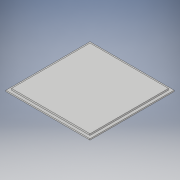
# Autodesk Inventor part: Boden
Saved by Autodesk Inventor 2018.3 (Build 223284000, 284)
## iProperties
Created: 2019-09-20
Part Number: Boden
Material: Generisch
Document SubType Name: Modeling
Designer: Lolob
Density: 1 g/cm^3
Appearance: Vorgabe
Author: Lolob
Autodesk Inventor part; units mm, degrees
ref_plane "YZ Plane" through (0, 0, 0) normal (1, 0, 0) x (0, 1, 0)
ref_plane "XZ Plane" through (0, 0, 0) normal (0, 1, 0) x (-1, 0, 0)
ref_plane "XY Plane" through (0, 0, 0) normal (0, 0, 1) x (1, 0, 0)
ref_plane "Arbeitsebene3" through (-858.9244, 0, 0) normal (0, 0, 1) x (1, 0, 0)
sketch "Skizze2" plane through (-858.9244, 0, 0) normal (0, 0, 1) x (1, 0, 0)
  line L0 (588.9244, 270) -> (1128.9244, 270)
  line L1 (1128.9244, 270) -> (1128.9244, -270)
  line L2 (1128.9244, -270) -> (588.9244, -270)
  line L3 (588.9244, -270) -> (588.9244, 270)
  line L4 (480.9244, 0) -> (1236.9244, 0) projected
  line L5 (858.9244, -378) -> (858.9244, 378) projected
  point P0 (858.9244, 0)
  dimension "d5" = 540
  dimension "d6" = 540
  constraints: 8 end point, 2 parallel, 1 horizontal, 1 perpendicular, 2 other
  measures "d5" distance of L0.start L0.end
  measures "d6" distance of L0.end L1.end
extrude "Extrusion2" add sketch "Skizze2" along normal blind 18
sketch "Skizze3" plane through (-858.9244, 0, 18) normal (0, 0, 1) x (1, 0, 0)
  line L0 (1128.9244, 270) -> (588.9244, 270) projected
  line L1 (588.9244, 270) -> (588.9244, -270) projected
  line L2 (588.9244, -270) -> (1128.9244, -270) projected
  line L3 (1128.9244, -270) -> (1128.9244, 270) projected
  line L4 (1110.9244, 252) -> (606.9244, 252)
  line L5 (606.9244, 252) -> (606.9244, -252)
  line L6 (606.9244, -252) -> (1110.9244, -252)
  line L7 (1110.9244, -252) -> (1110.9244, 252)
  point P0 (858.9244, 0)
  dimension "d12" = 18
  dimension "d13" = 18
  dimension "d14" = 18
  dimension "d15" = 18
  constraints: 8 end point, 2 parallel, 1 horizontal, 1 perpendicular
  measures "d12" distance between parallel lines of L0 L4
  measures "d13" distance between parallel lines of L3 L7
  measures "d14" distance between parallel lines of L2 L6
  measures "d15" distance between parallel lines of L1 L5
extrude "Extrusion3" cut sketch "Skizze3" against normal blind 10
